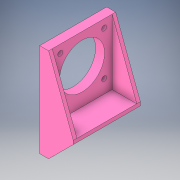
# Autodesk Inventor part: nemaMountStock
Saved by Autodesk Inventor 2019 (Build 230136000, 136)
## iProperties
Created: 2019-05-16
Part Number: nemaMountStock
Material: Generic
Document SubType Name: Modeling
Designer: Alex Jones
Density: 1 g/cm^3
Appearance: Default
Author: Alex Jones
Autodesk Inventor part; units mm, degrees
ref_plane "YZ Plane" through (0, 0, 0) normal (1, 0, 0) x (0, 1, 0)
ref_plane "XZ Plane" through (0, 0, 0) normal (0, 1, 0) x (-1, 0, 0)
ref_plane "XY Plane" through (0, 0, 0) normal (0, 0, 1) x (1, 0, 0)
sketch "Sketch2" plane through (0, 0, 0) normal (1, 0, 0) x (0, 1, 0)
  line L0 (-15.5, 15.5) -> (15.5, 15.5) construction
  line L1 (15.5, 15.5) -> (15.5, -15.5) construction
  line L2 (15.5, -15.5) -> (-15.5, -15.5) construction
  line L3 (-15.5, -15.5) -> (-15.5, 15.5) construction
  line L4 (-15.5, 15.5) -> (15.5, -15.5) construction
  line L5 (15.5, 15.5) -> (-15.5, -15.5) construction
  circle A0 centre (15.5, 15.5) radius 1.75
  circle A1 centre (15.5, -15.5) radius 1.75
  circle A2 centre (-15.5, -15.5) radius 1.75
  line L6 (-21.15, 21.15) -> (21.15, 21.15) construction
  line L7 (21.15, -21.15) -> (-21.15, -21.15) construction
  line L8 (-21.15, -21.15) -> (-21.15, 21.15) construction
  line L9 (-21.15, 21.15) -> (21.15, -21.15) construction
  line L10 (21.15, 21.15) -> (-21.15, -21.15) construction
  circle A3 centre (-15.5, 15.5) radius 1.75
  line L11 (21.15, 21.15) -> (-21.15, 21.15) construction
  line L12 (-21.15, 23.69) -> (21.15, 23.69)
  line L13 (21.15, -21.15) -> (-21.15, -21.15) construction
  line L14 (-21.15, -21.15) -> (-21.15, -23.69) construction
  line L15 (-21.15, -23.69) -> (21.15, -23.69)
  line L16 (-21.15, 21.15) -> (-44.96, 21.15) construction
  line L17 (-44.96, 21.15) -> (-44.96, -21.15)
  line L18 (-44.96, -21.15) -> (-21.15, -21.15) construction
  line L19 (-21.15, -21.15) -> (-21.15, 21.15) construction
  line L20 (-44.96, 21.15) -> (-20.6909, 21.15) construction
  line L21 (-44.96, -21.15) -> (-21.15, -21.15) construction
  line L22 (-34.96, 0.6795) -> (-34.96, -24.3695) construction
  line L23 (-34.96, 0.6795) -> (-34.96, 23.0105) construction
  circle A4 centre (-34.96, 11.845) radius 2.75
  circle A5 centre (-34.96, -11.845) radius 2.75
  circle A6 centre (0, 0) radius 15.875
  line L24 (-21.15, -23.69) -> (-24.96, -23.69)
  line L25 (-24.96, -23.69) -> (-24.96, 23.69) construction
  line L26 (-24.96, 23.69) -> (-21.15, 23.69)
  line L27 (-21.15, 23.69) -> (-21.15, -23.69) construction
  line L28 (21.15, -23.69) -> (21.15, 23.69)
  line L29 (21.15, -23.69) -> (-24.96, -23.69)
  line L30 (-24.96, -23.69) -> (-24.96, 23.69)
  line L31 (-24.96, 23.69) -> (21.15, 23.69)
  line L32 (21.15, 23.69) -> (21.15, -23.69)
  line L33 (-24.96, 23.69) -> (-44.96, 23.69)
  line L34 (-44.96, 23.69) -> (-44.96, -23.69)
  line L35 (-44.96, -23.69) -> (-24.96, -23.69)
  line L36 (-24.96, -23.69) -> (-24.96, 23.69)
  dimension "d19" = 31
  dimension "d20" = 3.5
  dimension "d21" = 42.3
  dimension "d24" = 5.5
  dimension "d35" = 31.75
  dimension "d36" = 23.69
  dimension "d38" = 20
  dimension "d39" = 42.3
  dimension "d40" = 3.81
  dimension "d41" = 10
  dimension "d42" = 2.54
  dimension "d43" = 42.3
  constraints: 74 end point, 13 parallel, 9 horizontal, 7 centre point, 7 perpendicular, 6 midpoint, 5 coincident, 4 equal radius, 2 collinear, 1 vertical
  measures "d19" distance of L0.end L1.end
  measures "d20" diameter of A1
  measures "d21" distance of L6.end L7.start
  measures "d24" diameter of A5
  measures "d35" diameter of A6
  measures "d36" distance of A4.centre A5.centre
  measures "d38" distance from line of L17 L24.end
  measures "d39" distance of L15.start L15.end
  measures "d40" distance of L15.start L24.end
  measures "d41" distance between parallel lines of L22 L17
  measures "d42" distance of L12.end L6.end
  measures "d43" distance of L12.start L12.end
extrude "Extrusion2" add sketch "Sketch2" along normal blind 6.35
sketch "Sketch3" plane through (6.35, 0, 0) normal (1, 0, 0) x (0, 0, -1)
  line L0 (-23.69, 21.15) -> (-23.69, -41.15) projected
  line L1 (-21.15, -44.96) -> (21.15, -44.96) projected
  line L2 (-23.69, 21.15) -> (-21.15, 21.15)
  line L3 (-21.15, 21.15) -> (-21.15, -44.96)
  line L4 (-21.15, -44.96) -> (-23.69, -44.96)
  line L5 (-23.69, -44.96) -> (-23.69, 21.15)
  line L6 (23.69, -24.96) -> (23.69, 21.15) projected
  line L7 (23.69, 21.15) -> (21.15, 21.15)
  line L8 (21.15, 21.15) -> (21.15, -44.96)
  line L9 (21.15, -44.96) -> (23.69, -44.96)
  line L10 (23.69, -44.96) -> (23.69, 21.15)
  line L11 (23.69, -27.5) -> (-23.69, -27.5)
  line L12 (-23.69, -27.5) -> (-23.69, -24.96)
  line L13 (-23.69, -24.96) -> (23.69, -24.96)
  line L14 (23.69, -24.96) -> (23.69, -27.5)
  point P0 (0, 0)
  point P1 (23.69, -41.15)
  dimension "d27" = 2.54
  dimension "d28" = 2.54
  dimension "d29" = 2.54
  dimension "d30" = 20
  constraints: 24 end point, 6 parallel, 3 horizontal, 3 perpendicular, 3 point on line, 2 other
  measures "d27" distance between parallel lines of L0 L3
  measures "d28" distance between parallel lines of L6 L8
  measures "d29" distance between parallel lines of L11 L13
extrude "Extrusion3" add sketch "Sketch3" along normal blind 17.46 contours L2 L3 L13 L0 | L13 L3 L11 L0 | L11 L3 L4 L5 L0 | L13 L8 L11 L3 | L13 L10 L11 L8 | L8 L7 L6 L13 | L11 L10 L9 L8
sketch "Sketch5" plane through (0, -44.96, 23.69) normal (0, 0, 1) x (1, 0, 0)
  line L0 (23.81, 20) -> (6.35, 20) projected
  line L1 (23.81, 66.11) -> (23.81, 20) projected
  line L2 (6.35, 66.11) -> (23.81, 66.11) projected
  line L3 (6.35, 20) -> (6.35, 66.11) projected
  line L4 (6.35, 17.46) -> (23.81, 17.46) projected
  line L5 (6.35, 0) -> (6.35, 17.46) projected
  line L6 (6.35, 0) -> (23.81, 0) projected
  line L7 (23.81, 17.46) -> (23.81, 0) projected
  line L8 (6.35, 0) -> (6.35, 17.46) projected
  line L9 (23.81, 17.46) -> (6.35, 0)
  line L10 (23.81, 20) -> (6.35, 66.11)
  point P0 (0, 44.96)
  constraints: 4 end point
extrude "Extrusion5" cut sketch "Sketch5" against normal through all contours L10 L2 L1 | L7 L6 L9
body "Solid2"
